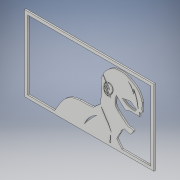
# Autodesk Inventor part: layer 4
Saved by Autodesk Inventor 2019 (Build 230136000, 136)
## iProperties
Created: 2018-11-19
Part Number: layer 4
Material: Generic
Document SubType Name: Modeling
Designer: Dajeh.white
Density: 1 g/cm^3
Appearance: Default
Author: Dajeh.white
Autodesk Inventor part; units mm, degrees
ref_plane "YZ Plane" through (0, 0, 0) normal (1, 0, 0) x (0, 1, 0)
ref_plane "XZ Plane" through (0, 0, 0) normal (0, 1, 0) x (-1, 0, 0)
ref_plane "XY Plane" through (0, 0, 0) normal (0, 0, 1) x (1, 0, 0)
sketch "Sketch1" plane through (0, 0, 0) normal (0, 0, 1) x (1, 0, 0)
  line L0 (0.0707, -1.4232) -> (254.0707, -1.4232) construction
  line L1 (254.0707, -1.4232) -> (254.0707, -144.2982) construction
  line L2 (254.0707, -144.2982) -> (0.0707, -144.2982) construction
  line L3 (0.0707, -144.2982) -> (0.0707, -1.4232) construction
  line L4 (-6.2793, 4.9268) -> (260.4207, 4.9268)
  line L5 (260.4207, 4.9268) -> (260.4207, -150.6482)
  line L6 (260.4207, -150.6482) -> (-6.2793, -150.6482)
  line L7 (-6.2793, -150.6482) -> (-6.2793, 4.9268)
  line L8 (0.0707, -1.4232) -> (254.0707, -1.4232)
  line L9 (254.0707, -1.4232) -> (254.0707, -144.2982)
  line L10 (0.0707, -144.4349) -> (0.0707, -1.4232)
  line L11 (194.4723, -144.2982) -> (185.184, -132.876) construction
  line L12 (185.184, -132.876) -> (185.0719, -132.7407) construction
  line L13 (185.0719, -132.7407) -> (183.9232, -130.2135) construction
  line L14 (183.9232, -130.2135) -> (184.2487, -129.0264) construction
  line L15 (184.2487, -129.0264) -> (186.6993, -124.3357) construction
  line L16 (186.6993, -124.3357) -> (186.661, -124.508) construction
  line L17 (186.661, -124.508) -> (189.0689, -119.9005) construction
  spline S0 degree 4 poles (194.4723, -144.2982) (185.184, -132.876) (185.0719, -132.7407) (183.9232, -130.2135) (184.2487, -129.0264) (186.6993, -124.3357) (186.661, -124.508) (189.0689, -119.9005) knots 1 1 1 1 1 2 3 4 5 5 5 5 5
  line L18 (189.0689, -119.9005) -> (192.3832, -114.3767) construction
  line L19 (192.3832, -114.3767) -> (193.0295, -112.3219) construction
  line L20 (193.0295, -112.3219) -> (192.8592, -111.4441) construction
  line L21 (192.8592, -111.4441) -> (193.0676, -111.2767) construction
  line L22 (193.0676, -111.2767) -> (194.8013, -109.4813) construction
  spline S1 degree 4 poles (189.0689, -119.9005) (192.3832, -114.3767) (193.0295, -112.3219) (192.8592, -111.4441) (193.0676, -111.2767) (194.8013, -109.4813) knots 1 1 1 1 1 2 3 3 3 3 3
  line L23 (194.8013, -109.4813) -> (199.1071, -105.4224) construction
  line L24 (199.1071, -105.4224) -> (199.4582, -105.1403) construction
  line L25 (199.4582, -105.1403) -> (200.3082, -105.1403) construction
  line L26 (200.3082, -105.1403) -> (209.1825, -108.7322) construction
  line L27 (209.1825, -108.7322) -> (209.3285, -108.9139) construction
  line L28 (209.3285, -108.9139) -> (210.9864, -108.5922) construction
  line L29 (210.9864, -108.5922) -> (213.5726, -108.0904) construction
  line L30 (213.5726, -108.0904) -> (214.5801, -104.9614) construction
  line L31 (214.5801, -104.9614) -> (217.8497, -101.1208) construction
  spline S2 degree 4 poles (194.8013, -109.4813) (199.1071, -105.4224) (199.4582, -105.1403) (200.3082, -105.1403) (209.1825, -108.7322) (209.3285, -108.9139) (210.9864, -108.5922) (213.5726, -108.0904) (214.5801, -104.9614) (217.8497, -101.1208) knots 1 1 1 1 1 2 3 4 5 6 7 7 7 7 7
  line L32 (217.8497, -101.1208) -> (218.4975, -99.8809) construction
  line L33 (218.4975, -99.8809) -> (218.6777, -99.2237) construction
  line L34 (218.6777, -99.2237) -> (218.3401, -98.8035) construction
  line L35 (218.3401, -98.8035) -> (218.3703, -98.8035) construction
  line L36 (218.3703, -98.8035) -> (217.8496, -99.1512) construction
  line L37 (217.8496, -99.1512) -> (214.7495, -97.2911) construction
  line L38 (214.7495, -97.2911) -> (214.0764, -97.1043) construction
  line L39 (214.0764, -97.1043) -> (210.9864, -97.1043) construction
  line L40 (210.9864, -97.1043) -> (208.0092, -97.682) construction
  line L41 (208.0092, -97.682) -> (206.598, -97.2656) construction
  line L42 (206.598, -97.2656) -> (199.2826, -91.0005) construction
  line L43 (199.2826, -91.0005) -> (185.8314, -79.3887) construction
  spline S3 degree 4 poles (217.8497, -101.1208) (218.4975, -99.8809) (218.6777, -99.2237) (218.3401, -98.8035) (218.3703, -98.8035) (217.8496, -99.1512) (214.7495, -97.2911) (214.0764, -97.1043) (210.9864, -97.1043) (208.0092, -97.682) (206.598, -97.2656) (199.2826, -91.0005) (185.8314, -79.3887) knots 1 1 1 1 1 2 3 4 5 6 7 8 9 10 10 10 10 10
  line L44 (185.8314, -79.3887) -> (181.8467, -75.0005) construction
  line L45 (181.8467, -75.0005) -> (181.1539, -72.474) construction
  line L46 (181.1539, -72.474) -> (180.4611, -68.4803) construction
  line L47 (180.4611, -68.4803) -> (181.2354, -61.4304) construction
  line L48 (181.2354, -61.4304) -> (182.621, -53.4431) construction
  line L49 (182.621, -53.4431) -> (182.6215, -53.4431) construction
  line L50 (182.6215, -53.4431) -> (185.637, -56.298) construction
  line L51 (185.637, -56.298) -> (201.8556, -70.9254) construction
  line L52 (201.8556, -70.9254) -> (202.1361, -70.9254) construction
  line L53 (202.1361, -70.9254) -> (204.3508, -69.946) construction
  line L54 (204.3508, -69.946) -> (207.0751, -68.108) construction
  line L55 (207.0751, -68.108) -> (209.4915, -67.6766) construction
  line L56 (209.4915, -67.6766) -> (213.3475, -67.1763) construction
  line L57 (213.3475, -67.1763) -> (217.4226, -67.5838) construction
  line L58 (217.4226, -67.5838) -> (220.605, -68.0743) construction
  line L59 (220.605, -68.0743) -> (226.8787, -66.8546) construction
  line L60 (226.8787, -66.8546) -> (229.243, -67.0717) construction
  line L61 (229.243, -67.0717) -> (229.6513, -68.105) construction
  line L62 (229.6513, -68.105) -> (230.1983, -68.7649) construction
  spline S4 degree 4 poles (185.8314, -79.3887) (181.8467, -75.0005) (181.1539, -72.474) (180.4611, -68.4803) (181.2354, -61.4304) (182.621, -53.4431) (182.6215, -53.4431) (185.637, -56.298) (201.8556, -70.9254) (202.1361, -70.9254) (204.3508, -69.946) (207.0751, -68.108) (209.4915, -67.6766) (213.3475, -67.1763) (217.4226, -67.5838) (220.605, -68.0743) (226.8787, -66.8546) (229.243, -67.0717) (229.6513, -68.105) (230.1983, -68.7649) knots 1 1 1 1 1 2 3 4 5 6 7 8 9 10 11 12 13 14 15 16 17 17 17 17 17
  line L63 (230.1983, -68.7649) -> (230.5913, -68.5281) construction
  line L64 (230.5913, -68.5281) -> (231.0087, -68.0642) construction
  line L65 (231.0087, -68.0642) -> (230.4579, -65.2257) construction
  line L66 (230.4579, -65.2257) -> (229.721, -61.6152) construction
  line L67 (229.721, -61.6152) -> (230.0353, -60.3215) construction
  line L68 (230.0353, -60.3215) -> (230.5632, -59.706) construction
  line L69 (230.5632, -59.706) -> (230.536, -59.706) construction
  line L70 (230.536, -59.706) -> (233.5475, -60.4834) construction
  line L71 (233.5475, -60.4834) -> (234.3033, -60.1758) construction
  line L72 (234.3033, -60.1758) -> (236.4483, -58.0018) construction
  line L73 (236.4483, -58.0018) -> (236.0714, -54.5553) construction
  line L74 (236.0714, -54.5553) -> (235.9378, -54.1446) construction
  line L75 (235.9378, -54.1446) -> (234.7256, -51.4381) construction
  line L76 (234.7256, -51.4381) -> (235.9378, -50.8952) construction
  line L77 (235.9378, -50.8952) -> (236.0766, -44.4647) construction
  line L78 (236.0766, -44.4647) -> (236.3701, -41.064) construction
  spline S5 degree 4 poles (230.1983, -68.7649) (230.5913, -68.5281) (231.0087, -68.0642) (230.4579, -65.2257) (229.721, -61.6152) (230.0353, -60.3215) (230.5632, -59.706) (230.536, -59.706) (233.5475, -60.4834) (234.3033, -60.1758) (236.4483, -58.0018) (236.0714, -54.5553) (235.9378, -54.1446) (234.7256, -51.4381) (235.9378, -50.8952) (236.0766, -44.4647) (236.3701, -41.064) knots 1 1 1 1 1 2 3 4 5 6 7 8 9 10 11 12 13 14 14 14 14 14
  line L79 (236.3701, -41.064) -> (235.052, -34.1465) construction
  line L80 (235.052, -34.1465) -> (229.7334, -24.5357) construction
  line L81 (229.7334, -24.5357) -> (226.5609, -20.8966) construction
  line L82 (226.5609, -20.8966) -> (222.4382, -17.4275) construction
  line L83 (222.4382, -17.4275) -> (208.2833, -8.9923) construction
  line L84 (208.2833, -8.9923) -> (201.8556, -7.1634) construction
  line L85 (201.8556, -7.1634) -> (194.8013, -5.2804) construction
  line L86 (194.8013, -5.2804) -> (182.6215, -7.0364) construction
  line L87 (182.6215, -7.0364) -> (178.104, -7.0364) construction
  line L88 (178.104, -7.0364) -> (167.9672, -13.8036) construction
  line L89 (152.7647, -36.8927) -> (151.3863, -40.2982) construction
  line L90 (151.3863, -40.2982) -> (151.237, -45.8507) construction
  line L91 (151.237, -45.8507) -> (152.7804, -56.2786) construction
  line L92 (152.7804, -56.2786) -> (153.5939, -60.1758) construction
  line L93 (153.5939, -60.1758) -> (153.0487, -61.9022) construction
  line L94 (153.0487, -61.9022) -> (149.9019, -85.8619) construction
  spline S6 degree 4 poles (151.3863, -40.2982) (151.237, -45.8507) (152.7804, -56.2786) (153.5939, -60.1758) (153.0487, -61.9022) (149.9019, -85.8619) knots 1 1 1 1 1 2 3 3 3 3 3
  line L95 (149.9019, -85.8619) -> (136.5549, -97.682) construction
  line L96 (136.5549, -97.682) -> (136.2912, -98.4107) construction
  line L97 (136.2912, -98.4107) -> (133.5401, -98.4941) construction
  line L98 (133.5401, -98.4941) -> (132.4564, -99.3277) construction
  line L99 (132.4564, -99.3277) -> (126.7875, -99.8279) construction
  line L100 (126.7875, -99.8279) -> (107.9468, -100.3281) construction
  spline S7 degree 4 poles (149.9019, -85.8619) (136.5549, -97.682) (136.2912, -98.4107) (133.5401, -98.4941) (132.4564, -99.3277) (126.7875, -99.8279) (107.9468, -100.3281) knots 1 1 1 1 1 2 3 4 4 4 4 4
  line L101 (195.4344, -52.7913) -> (205.0695, -50.2291) construction
  line L102 (205.0695, -50.2291) -> (211.9395, -49.1447) construction
  line L103 (211.9395, -49.1447) -> (213.5056, -50.1155) construction
  line L104 (213.5056, -50.1155) -> (216.6138, -52.7546) construction
  line L105 (216.6138, -52.7546) -> (218.9596, -54.5726) construction
  line L106 (218.9596, -54.5726) -> (221.0708, -55.5109) construction
  line L107 (221.0708, -55.5109) -> (224.6482, -57.5635) construction
  line L108 (224.6482, -57.5635) -> (224.9414, -58.3258) construction
  line L109 (224.9414, -58.3258) -> (221.7746, -63.1347) construction
  line L110 (221.7746, -63.1347) -> (219.8979, -63.1347) construction
  line L111 (219.8979, -63.1347) -> (206.0577, -59.9093) construction
  line L112 (206.0577, -59.9093) -> (205.354, -60.1438) construction
  line L113 (205.354, -60.1438) -> (195.4344, -52.7913) construction
  spline S8 degree 4 poles (195.4344, -52.7913) (205.0695, -50.2291) (211.9395, -49.1447) (213.5056, -50.1155) (216.6138, -52.7546) (218.9596, -54.5726) (221.0708, -55.5109) (224.6482, -57.5635) (224.9414, -58.3258) (221.7746, -63.1347) (219.8979, -63.1347) (206.0577, -59.9093) (205.354, -60.1438) (195.4344, -52.7913) knots 1 1 1 1 1 2 3 4 5 6 7 8 9 10 11 11 11 11 11
  line L114 (227.7208, -55.3149) -> (227.1106, -49.5793) construction
  line L115 (227.1106, -49.5793) -> (223.1445, -34.8131) construction
  line L116 (223.1445, -34.8131) -> (219.6665, -26.8808) construction
  line L117 (219.6665, -26.8808) -> (219.6055, -26.5757) construction
  line L118 (219.6055, -26.5757) -> (219.7275, -28.1012) construction
  line L119 (219.7275, -28.1012) -> (219.2394, -34.2639) construction
  line L120 (219.2394, -34.2639) -> (218.7512, -34.2639) construction
  line L121 (218.7512, -34.2639) -> (217.836, -31.9453) construction
  line L122 (217.836, -31.9453) -> (214.3758, -23.1796) construction
  line L123 (214.3758, -23.1796) -> (207.402, -16.7519) construction
  spline S9 degree 4 poles (227.7208, -55.3149) (227.1106, -49.5793) (223.1445, -34.8131) (219.6665, -26.8808) (219.6055, -26.5757) (219.7275, -28.1012) (219.2394, -34.2639) (218.7512, -34.2639) (217.836, -31.9453) (214.3758, -23.1796) (207.402, -16.7519) knots 1 1 1 1 1 2 3 4 5 6 7 8 8 8 8 8
  line L124 (207.402, -16.7519) -> (213.1424, -20.6706) construction
  line L125 (213.1424, -20.6706) -> (216.4663, -25.6564) construction
  line L126 (216.4663, -25.6564) -> (218.6822, -30.827) construction
  line L127 (218.6822, -30.827) -> (218.6822, -31.1963) construction
  line L128 (218.6822, -31.1963) -> (218.6822, -25.3795) construction
  line L129 (218.6822, -25.3795) -> (218.5899, -23.7175) construction
  line L130 (218.5899, -23.7175) -> (218.7745, -24.1792) construction
  line L131 (218.7745, -24.1792) -> (224.222, -33.5045) construction
  line L132 (224.222, -33.5045) -> (226.5303, -42.9223) construction
  spline S10 degree 4 poles (207.402, -16.7519) (213.1424, -20.6706) (216.4663, -25.6564) (218.6822, -30.827) (218.6822, -31.1963) (218.6822, -25.3795) (218.5899, -23.7175) (218.7745, -24.1792) (224.222, -33.5045) (226.5303, -42.9223) knots 1 1 1 1 1 2 3 4 5 6 7 7 7 7 7
  line L133 (226.5303, -42.9223) -> (228.0805, -51.8862) construction
  line L134 (228.0805, -51.8862) -> (227.7208, -55.3149) construction
  spline S11 degree 2 poles (226.5303, -42.9223) (228.0805, -51.8862) (227.7208, -55.3149) knots 1 1 1 2 2 2
  line L135 (155.7412, -29.539) -> (164.0298, -41.2857) construction
  line L136 (164.0298, -41.2857) -> (169.665, -49.8323) construction
  line L137 (169.665, -49.8323) -> (169.7119, -49.8323) construction
  line L138 (169.7119, -49.8323) -> (169.7119, -50.3019) construction
  line L139 (169.7119, -50.3019) -> (163.842, -50.3019) construction
  line L140 (163.842, -50.3019) -> (163.842, -50.3958) construction
  line L141 (163.842, -50.3958) -> (163.7481, -50.3958) construction
  line L142 (163.7481, -50.3958) -> (171.4025, -63.4505) construction
  line L143 (171.4025, -63.4505) -> (171.4494, -63.8731) construction
  line L144 (171.4494, -63.8731) -> (171.5903, -63.9671) construction
  line L145 (171.5903, -63.9671) -> (166.6596, -61.6661) construction
  line L146 (166.6596, -61.6661) -> (159.0991, -57.2519) construction
  line L147 (159.0991, -57.2519) -> (158.9113, -56.8762) construction
  line L148 (158.9113, -56.8762) -> (158.9582, -56.5944) construction
  line L149 (158.9582, -56.5944) -> (165.6734, -59.7407) construction
  line L150 (165.6734, -59.7407) -> (165.7673, -59.5529) construction
  line L151 (165.7673, -59.5529) -> (162.668, -55.4674) construction
  line L152 (162.668, -55.4674) -> (157.5494, -46.8269) construction
  line L153 (157.5494, -46.8269) -> (156.7981, -46.0286) construction
  line L154 (156.7981, -46.0286) -> (156.7511, -45.512) construction
  line L155 (156.7511, -45.512) -> (165.2038, -47.5313) construction
  line L156 (165.2038, -47.5313) -> (165.016, -47.2026) construction
  line L157 (165.016, -47.2026) -> (160.7896, -39.8299) construction
  line L158 (160.7896, -39.8299) -> (155.3423, -30.5789) construction
  line L159 (155.3423, -30.5789) -> (155.2628, -30.6623) construction
  spline S12 degree 4 poles (155.7412, -29.539) (164.0298, -41.2857) (169.665, -49.8323) (169.7119, -49.8323) (169.7119, -50.3019) (163.842, -50.3019) (163.842, -50.3958) (163.7481, -50.3958) (171.4025, -63.4505) (171.4494, -63.8731) (171.5903, -63.9671) (166.6596, -61.6661) (159.0991, -57.2519) (158.9113, -56.8762) (158.9582, -56.5944) (165.6734, -59.7407) (165.7673, -59.5529) (162.668, -55.4674) (157.5494, -46.8269) (156.7981, -46.0286) (156.7511, -45.512) (165.2038, -47.5313) (165.016, -47.2026) (160.7896, -39.8299) (155.3423, -30.5789) (155.2628, -30.6623) knots 1 1 1 1 1 2 3 4 5 6 7 8 9 10 11 12 13 14 15 16 17 18 19 20 21 22 23 23 23 23 23
  line L160 (168.5837, -39.9518) -> (170.8025, -40.3434) construction
  line L161 (170.8025, -40.3434) -> (172.4991, -41.1699) construction
  line L162 (172.4991, -41.1699) -> (173.8043, -42.3011) construction
  line L163 (173.8043, -42.3011) -> (174.5873, -43.6062) construction
  line L164 (174.5873, -43.6062) -> (175.2739, -46.3094) construction
  spline S13 degree 4 poles (168.5837, -39.9518) (170.8025, -40.3434) (172.4991, -41.1699) (173.8043, -42.3011) (174.5873, -43.6062) (175.2739, -46.3094) (175.0736, -49.7843) (173.8256, -53.3106) (170.1467, -58.4696) knots 1 1 1 1 1 2 3 4 5 5.945096 5.945096 5.945096 5.945096 5.945096
  line L165 (168.5837, -39.9518) -> (167.5858, -39.96) construction
  spline S14 degree 2 poles (168.5837, -39.9518) (167.5858, -39.96) (166.2437, -40.1778) knots 1 1 1 1.534366 1.534366 1.534366
  line L166 (162.1665, -62.1538) -> (160.458, -61.073) construction
  line L167 (160.458, -61.073) -> (159.1791, -58.977) construction
  spline S15 degree 4 poles (165.3844, -62.331) (164.6941, -62.5961) (163.5161, -62.659) (162.1665, -62.1538) (160.458, -61.073) (159.1791, -58.977) (158.3997, -56.3708) (158.0862, -52.2088) (158.1975, -50.3279) knots 1.278391 1.278391 1.278391 1.278391 1.278391 2 3 4 5 5.791918 5.791918 5.791918 5.791918 5.791918
  spline S16 degree 2 poles (159.6396, -45.1633) (160.4077, -44.0591) (161.3972, -42.6367) knots 1.269112 1.269112 1.269112 1.850767 1.850767 1.850767
  line L168 (171.2746, -38.6806) -> (173.0121, -39.7498) construction
  line L169 (173.0121, -39.7498) -> (175.7477, -42.8602) construction
  line L170 (175.7477, -42.8602) -> (177.1849, -46.9136) construction
  spline S17 degree 4 poles (165.2708, -38.645) (166.2643, -38.5317) (168.9548, -38.35) (171.2746, -38.6806) (173.0121, -39.7498) (175.7477, -42.8602) (177.1849, -46.9136) (176.7072, -50.6709) (174.2827, -55.5383) (171.1296, -59.8511) knots 1.433621 1.433621 1.433621 1.433621 1.433621 2 3 4 5 6 6.933225 6.933225 6.933225 6.933225 6.933225
  spline S18 degree 4 poles (160.3746, -41.2567) (159.9642, -41.9468) (159.467, -42.7604) (158.9971, -43.7224) (158.5885, -44.7526) knots 1.241216 1.241216 1.241216 1.241216 1.241216 1.829723 1.829723 1.829723 1.829723 1.829723
  line L171 (160.9264, -40.2396) -> (160.9568, -40.1689) construction
  spline S19 degree 1 poles (160.9264, -40.2396) (160.9568, -40.1689) knots 1 1 2 2
  line L172 (161.9195, -41.8859) -> (161.9382, -41.8591) construction
  spline S20 degree 1 poles (161.9195, -41.8859) (161.9382, -41.8591) knots 1 1 2 2
  line L173 (162.4817, -39.1502) -> (162.465, -39.1553) construction
  spline S21 degree 1 poles (162.4817, -39.1502) (162.465, -39.1553) knots 1 1 2 2
  line L174 (163.6434, -40.7166) -> (163.556, -40.7379) construction
  spline S22 degree 1 poles (163.6434, -40.7166) (163.556, -40.7379) knots 1 1 2 2
  line L175 (169.2273, -59.7407) -> (169.2132, -59.76) construction
  spline S23 degree 1 poles (169.2273, -59.7407) (169.2132, -59.76) knots 1 1 2 2
  line L176 (156.8902, -51.5462) -> (156.8902, -51.7633) construction
  spline S24 degree 4 poles (157.1034, -49.4022) (156.9707, -50.3993) (156.8967, -51.1312) (156.8902, -51.5462) (156.8902, -51.7633) knots 1.338614 1.338614 1.338614 1.338614 1.338614 2 2 2 2 2
  line L177 (160.6702, -62.2927) -> (158.8281, -60.4506) construction
  line L178 (158.8281, -60.4506) -> (157.1394, -56.5784) construction
  line L179 (157.1394, -56.5784) -> (156.7318, -53.5797) construction
  line L180 (156.7318, -53.5797) -> (156.8902, -51.7633) construction
  spline S25 degree 4 poles (166.8937, -63.2493) (165.2569, -63.5103) (162.5673, -63.2416) (160.6702, -62.2927) (158.8281, -60.4506) (157.1394, -56.5784) (156.7318, -53.5797) (156.8902, -51.7633) knots 1.222653 1.222653 1.222653 1.222653 1.222653 2 3 4 5 5 5 5 5
  line L181 (157.4581, -46.9824) -> (157.4727, -46.8991) construction
  spline S26 degree 1 poles (157.4581, -46.9824) (157.4727, -46.8991) knots 1 1 2 2
  line L182 (107.9468, -100.3281) -> (95.0504, -101.8958) construction
  line L183 (95.0504, -101.8958) -> (86.4127, -105.1042) construction
  line L184 (86.4127, -105.1042) -> (77.1505, -112.1726) construction
  spline S27 degree 4 poles (107.9468, -100.3281) (95.0504, -101.8958) (86.4127, -105.1042) (77.1505, -112.1726) (71.0178, -119.2411) (66.436, -126.6459) (55.7989, -144.4349) knots 1 1 1 1 1 2 3 3.962899 3.962899 3.962899 3.962899 3.962899
  line L185 (77.1505, -112.1726) -> (71.0178, -119.2411) construction
  line L186 (71.0178, -119.2411) -> (66.436, -126.6459) construction
  line L187 (66.436, -126.6459) -> (55.7989, -144.4349) construction
  line L188 (171.4723, -144.4349) -> (171.6641, -139.8547) construction
  line L189 (171.6641, -139.8547) -> (171.5746, -134.8418) construction
  line L190 (171.5746, -134.8418) -> (171.7536, -131.0821) construction
  line L191 (171.7536, -131.0821) -> (170.0528, -129.9184) construction
  line L192 (170.0528, -129.9184) -> (170.1543, -134.2051) construction
  spline S28 degree 4 poles (171.4723, -144.4349) (171.6641, -139.8547) (171.5746, -134.8418) (171.7536, -131.0821) (170.0528, -129.9184) (170.1543, -134.2051) (170.1551, -136.3472) (169.8627, -138.7923) (169.7948, -144.4349) knots 1 1 1 1 1 2 3 4 5 5.966145 5.966145 5.966145 5.966145 5.966145
  line L193 (170.1543, -134.2051) -> (170.1551, -136.3472) construction
  line L194 (170.1551, -136.3472) -> (169.8627, -138.7923) construction
  line L195 (169.8627, -138.7923) -> (169.7948, -144.4349) construction
  line L196 (254.0707, -144.2982) -> (194.4723, -144.2982)
  line L197 (151.7288, -89.7379) -> (154.695, -92.9039) construction
  line L198 (154.695, -92.9039) -> (156.9489, -96.4726) construction
  line L199 (156.9489, -96.4726) -> (159.5159, -100.6362) construction
  line L200 (159.5159, -100.6362) -> (161.3629, -104.0796) construction
  line L201 (161.3629, -104.0796) -> (165.6536, -109.5385) construction
  line L202 (165.6536, -109.5385) -> (165.5185, -109.6061) construction
  line L203 (165.5185, -109.6061) -> (167.9508, -114.2342) construction
  line L204 (167.9508, -114.2342) -> (169.8426, -117.7476) construction
  line L205 (169.8426, -117.7476) -> (172.6184, -124.7951) construction
  spline S29 degree 4 poles (151.7288, -89.7379) (154.695, -92.9039) (156.9489, -96.4726) (159.5159, -100.6362) (161.3629, -104.0796) (165.6536, -109.5385) (165.5185, -109.6061) (167.9508, -114.2342) (169.8426, -117.7476) (172.6184, -124.7951) knots 1 1 1 1 1 2 3 4 5 6 7 7 7 7 7
  line L206 (172.6184, -124.7951) -> (170.6471, -121.528) construction
  line L207 (170.6471, -121.528) -> (169.2556, -118.6953) construction
  line L208 (169.2556, -118.6953) -> (168.0131, -115.7797) construction
  line L209 (168.0131, -115.7797) -> (167.1683, -114.6201) construction
  line L210 (167.1683, -114.6201) -> (164.6928, -110.7183) construction
  line L211 (164.6928, -110.7183) -> (161.4532, -106.3281) construction
  line L212 (161.4532, -106.3281) -> (158.9099, -102.3315) construction
  line L213 (158.9099, -102.3315) -> (156.3363, -97.8202) construction
  line L214 (156.3363, -97.8202) -> (154.6408, -95.0953) construction
  line L215 (154.6408, -95.0953) -> (152.9817, -92.1982) construction
  line L216 (152.9817, -92.1982) -> (151.7288, -89.7379) construction
  spline S30 degree 4 poles (172.6184, -124.7951) (170.6471, -121.528) (169.2556, -118.6953) (168.0131, -115.7797) (167.1683, -114.6201) (164.6928, -110.7183) (161.4532, -106.3281) (158.9099, -102.3315) (156.3363, -97.8202) (154.6408, -95.0953) (152.9817, -92.1982) (151.7288, -89.7379) knots 1 1 1 1 1 2 3 4 5 6 7 8 9 9 9 9 9
  line L217 (142.3099, -109.6061) -> (135.7764, -116.3224) construction
  line L218 (135.7764, -116.3224) -> (128.6964, -123.2001) construction
  line L219 (128.6964, -123.2001) -> (122.8301, -130.1789) construction
  line L220 (122.8301, -130.1789) -> (119.6947, -134.0224) construction
  line L221 (119.6947, -134.0224) -> (116.8627, -137.8658) construction
  spline S31 degree 4 poles (142.3099, -109.6061) (135.7764, -116.3224) (128.6964, -123.2001) (122.8301, -130.1789) (119.6947, -134.0224) (116.8627, -137.8658) knots 1 1 1 1 1 2 3 3 3 3 3
  line L222 (116.8627, -137.8658) -> (119.7958, -130.6847) construction
  line L223 (119.7958, -130.6847) -> (124.6507, -123.7058) construction
  line L224 (124.6507, -123.7058) -> (130.1124, -117.1315) construction
  line L225 (130.1124, -117.1315) -> (137.2935, -112.1756) construction
  line L226 (137.2935, -112.1756) -> (142.3099, -109.6061) construction
  spline S32 degree 4 poles (116.8627, -137.8658) (119.7958, -130.6847) (124.6507, -123.7058) (130.1124, -117.1315) (137.2935, -112.1756) (142.3099, -109.6061) knots 1 1 1 1 1 2 3 3 3 3 3
  line L227 (171.4723, -144.4349) -> (169.7948, -144.4349)
  line L228 (55.7989, -144.4349) -> (0.0707, -144.4349)
  spline S33 degree 4 poles (236.3701, -41.064) (235.052, -34.1465) (229.7334, -24.5357) (226.5609, -20.8966) (222.4382, -17.4275) (208.2833, -8.9923) (201.8556, -7.1634) (194.8013, -5.2804) (182.6215, -7.0364) (178.104, -7.0364) (167.9672, -13.8036) (159.5051, -22.2341) (157.0238, -26.5922) (155.7412, -29.539) knots 1 1 1 1 1 2 3 4 5 6 7 8 9 10 10.631148 10.631148 10.631148 10.631148 10.631148
  spline S34 degree 4 poles (155.2628, -30.6623) (154.5762, -32.305) (153.7766, -34.3202) (152.7647, -36.8927) (151.3863, -40.2982) knots 0 0 0 0 0 1 1 1 1 1
  line L229 (167.9672, -13.8036) -> (159.5051, -22.2341) construction
  line L230 (159.5051, -22.2341) -> (157.0238, -26.5922) construction
  line L231 (157.0238, -26.5922) -> (155.7412, -29.539) construction
  line L232 (153.7766, -34.3202) -> (152.7647, -36.8927) construction
  line L233 (154.5762, -32.305) -> (153.7766, -34.3202) construction
  line L234 (155.2628, -30.6623) -> (154.5762, -32.305) construction
  line L235 (165.2708, -38.645) -> (166.2437, -40.1778)
  line L236 (165.2708, -38.645) -> (166.2643, -38.5317) construction
  line L237 (166.2643, -38.5317) -> (168.9548, -38.35) construction
  line L238 (168.9548, -38.35) -> (171.2746, -38.6806) construction
  line L239 (167.5858, -39.96) -> (166.2437, -40.1778) construction
  line L240 (170.1467, -58.4696) -> (171.1296, -59.8511)
  line L241 (175.2739, -46.3094) -> (175.0736, -49.7843) construction
  line L242 (175.0736, -49.7843) -> (173.8256, -53.3106) construction
  line L243 (173.8256, -53.3106) -> (170.1467, -58.4696) construction
  line L244 (177.1849, -46.9136) -> (176.7072, -50.6709) construction
  line L245 (176.7072, -50.6709) -> (174.2827, -55.5383) construction
  line L246 (174.2827, -55.5383) -> (171.1296, -59.8511) construction
  line L247 (165.3844, -62.331) -> (166.8937, -63.2493)
  line L248 (165.3844, -62.331) -> (164.6941, -62.5961) construction
  line L249 (164.6941, -62.5961) -> (163.5161, -62.659) construction
  line L250 (163.5161, -62.659) -> (162.1665, -62.1538) construction
  line L251 (166.8937, -63.2493) -> (165.2569, -63.5103) construction
  line L252 (165.2569, -63.5103) -> (162.5673, -63.2416) construction
  line L253 (162.5673, -63.2416) -> (160.6702, -62.2927) construction
  line L254 (160.3746, -41.2567) -> (161.3972, -42.6367)
  line L255 (158.5885, -44.7526) -> (159.6396, -45.1633)
  line L256 (158.9971, -43.7224) -> (158.5885, -44.7526) construction
  line L257 (159.6396, -45.1633) -> (160.4077, -44.0591) construction
  line L258 (160.4077, -44.0591) -> (161.3972, -42.6367) construction
  line L259 (160.3746, -41.2567) -> (159.9642, -41.9468) construction
  line L260 (159.9642, -41.9468) -> (159.467, -42.7604) construction
  line L261 (159.467, -42.7604) -> (158.9971, -43.7224) construction
  line L262 (157.1034, -49.4022) -> (158.1975, -50.3279)
  line L263 (157.1034, -49.4022) -> (156.9707, -50.3993) construction
  line L264 (156.9707, -50.3993) -> (156.8967, -51.1312) construction
  line L265 (156.8967, -51.1312) -> (156.8902, -51.5462) construction
  line L266 (159.1791, -58.977) -> (158.3997, -56.3708) construction
  line L267 (158.3997, -56.3708) -> (158.0862, -52.2088) construction
  line L268 (158.0862, -52.2088) -> (158.1975, -50.3279) construction
  point P0 (0, 0)
  point P1 (0, 0)
  dimension "d5" = 254
  dimension "d9" = 6.35
  dimension "d11" = 6.35
  dimension "d12" = 6.35
  dimension "d13" = 6.35
  constraints: 32 end point, 9 horizontal, 6 parallel, 3 point on line, 2 perpendicular, 1 vertical, 112 other
  measures "d5" distance of L0.start L0.end
  measures "d9" distance between parallel lines of L1 L5
  measures "d11" distance between parallel lines of L3 L7
  measures "d12" distance between parallel lines of L6 L2
  measures "d13" distance between parallel lines of L4 L0
extrude "Extrusion1" add sketch "Sketch1" along normal blind 3.175
body "Solid1"
